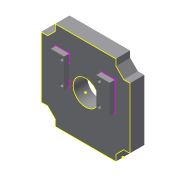
# Autodesk Inventor part: 20_Cube_Insert_RaspiCam_v3
Saved by Autodesk Inventor 2019.4 (Build 234330000, 330)
## iProperties
Created: 2019-07-01
Part Number: 20_Cube_Insert_RaspiCam_v3
Material: Generic
Document SubType Name: Modeling
Designer: diederichbenedict
Density: 1 g/cm^3
Appearance: Default
Author: diederichbenedict
Autodesk Inventor part; units mm, degrees
ref_plane "YZ Plane" through (0, 0, 0) normal (1, 0, 0) x (0, 1, 0)
ref_plane "Work Plane1" through (0, 0, 10) normal (0, 0, 1) x (1, 0, 0)
sketch "Sketch1" plane through (0, 0, 10) normal (0, 0, 1) x (1, 0, 0)
  line L0 (-4.0299, -0.3538) -> (-2.2322, 1.4439) construction
  arc A0 (-1.4439, 2.2322) -> (-2.2322, 1.4439) centre (-0.9299, 0.9299) ccw construction
  line L1 (-1.4439, 2.2322) -> (0.3538, 4.0299) construction
  line L2 (-37.8299, 42.2137) -> (-37.8299, 45.8299) construction
  line L3 (-37.8299, 45.8299) -> (-4.0299, 45.8299) construction
  line L4 (-4.0299, 45.8299) -> (-4.0299, 42.2137) construction
  line L5 (-4.0299, 4.0299) -> (0.3538, 4.0299) projected
  circle A1 centre (-20.9299, 20.9299) radius 17.5 projected
  line L6 (-20.9299, 58.9723) -> (17.1124, 20.9299) construction
  line L7 (17.1124, 20.9299) -> (-20.9299, -17.1124) construction
  line L8 (-20.9299, -17.1124) -> (-58.9723, 20.9299) construction
  line L9 (-58.9723, 20.9299) -> (-20.9299, 58.9723) construction
  line L10 (-20.9299, 58.9723) -> (-20.9299, -17.1124) construction
  line L11 (17.1124, 20.9299) -> (-58.9723, 20.9299) construction
  line L12 (-20.9299, 58.9723) -> (32.8701, 58.9723) construction
  line L13 (-43.4299, 43.4299) -> (1.5701, 43.4299) construction
  line L14 (1.5701, 43.4299) -> (1.5701, -1.5701) construction
  line L15 (1.5701, -1.5701) -> (-43.4299, -1.5701) construction
  line L16 (-43.4299, -1.5701) -> (-43.4299, 43.4299) construction
  line L17 (-43.4299, 43.4299) -> (1.5701, -1.5701) construction
  line L18 (1.5701, 43.4299) -> (-43.4299, -1.5701) construction
  line L19 (-43.4299, 5.3876) -> (-43.4299, 36.4723)
  line L20 (-43.4299, 36.4723) -> (-36.4723, 43.4299)
  line L21 (-36.4723, 43.4299) -> (-5.3876, 43.4299)
  line L22 (-5.3876, 43.4299) -> (1.5701, 36.4723)
  line L23 (1.5701, 36.4723) -> (1.5701, 5.3876)
  line L24 (1.5701, 5.3876) -> (-5.3876, -1.5701)
  line L25 (-5.3876, -1.5701) -> (-36.4723, -1.5701)
  line L26 (-36.4723, -1.5701) -> (-43.4299, 5.3876)
  line L27 (-4.0299, 42.2137) -> (-37.8299, 42.2137) projected
  line L28 (-4.0299, -0.3538) -> (-4.0299, 4.0299) projected
  circle A2 centre (-20.9299, 20.9299) radius 7.0417
  point P0 (-37.8299, 4.0299)
  dimension "d18" = 53.8
  dimension "d19" = 45
  dimension "d20" = 53.8
  dimension "d21" = 45
  dimension "d22" = 45
  constraints: 42 end point, 15 point on line, 5 midpoint, 4 parallel, 3 perpendicular, 2 horizontal, 1 centre point, 1 coincident, 1 equal length
  measures "d18" distance of L6.start L6.end
  measures "d19" angle of L6 L12
  measures "d20" distance of L6.end L7.end
  measures "d21" distance of L14.end L15.end
  measures "d22" distance of L13.end L14.end
extrude "Extrusion1" add sketch "Sketch1" along normal blind 8 contours L28 L24 L25 L26 L19 L20 L27 L22 L23 L5 | L5 L24 L28 | L27 L20 L21 L22 | A1
sketch "Sketch3" plane through (0, 0, 10) normal (0, 0, -1) x (-1, 0, 0)
  line L0 (37.8299, -0.4701) -> (37.8299, 4.0299) construction
  line L1 (4.0299, 4.0299) -> (4.0299, -0.4701) construction
  line L2 (37.8299, -0.4701) -> (37.8299, 1.1886) construction
  line L3 (4.0299, -3.9701) -> (4.0299, -0.3538) construction
  line L4 (45.8299, 4.0299) -> (42.2137, 4.0299) construction
  line L5 (-0.3538, 4.0299) -> (-3.9701, 4.0299) construction
  line L6 (-3.9701, 37.8299) -> (-0.3538, 37.8299) construction
  line L7 (4.0299, 42.2137) -> (4.0299, 45.8299) construction
  line L8 (37.8299, 45.8299) -> (37.8299, 42.2137) construction
  line L9 (42.2137, 37.8299) -> (45.8299, 37.8299) construction
  line L10 (37.8299, 37.7299) -> (45.8299, 37.7299)
  line L11 (45.8299, 37.7299) -> (45.8299, 4.1299)
  line L12 (45.8299, 4.1299) -> (37.8299, 4.1299)
  line L13 (37.8299, 4.1299) -> (37.8299, 37.7299)
  line L14 (37.7299, 4.0299) -> (4.1299, 4.0299)
  line L15 (4.1299, 4.0299) -> (4.1299, -3.9701)
  line L16 (4.1299, -3.9701) -> (37.7299, -3.9701)
  line L17 (37.7299, -3.9701) -> (37.7299, 4.0299)
  line L18 (4.0299, 4.1299) -> (-3.9701, 4.1299)
  line L19 (-3.9701, 4.1299) -> (-3.9701, 37.7299)
  line L20 (-3.9701, 37.7299) -> (4.0299, 37.7299)
  line L21 (4.0299, 37.7299) -> (4.0299, 4.1299)
  line L22 (4.1299, 37.8299) -> (37.7299, 37.8299)
  line L23 (37.7299, 37.8299) -> (37.7299, 45.8299)
  line L24 (37.7299, 45.8299) -> (4.1299, 45.8299)
  line L25 (4.1299, 45.8299) -> (4.1299, 37.8299)
  point P0 (0, 0)
  dimension "d23" = 0.1
  dimension "d24" = 0.1
  dimension "d25" = 0.1
  dimension "d26" = 0.1
  dimension "d27" = 0.1
  constraints: 32 end point, 8 parallel, 4 horizontal, 4 perpendicular, 3 point on line
  measures "d23" distance between parallel lines of L8 L23
  measures "d24" distance between parallel lines of L7 L25
  measures "d25" distance between parallel lines of L6 L20
  measures "d26" distance between parallel lines of L5 L18
  measures "d27" distance between parallel lines of L1 L15
extrude "Extrusion3" add sketch "Sketch3" against normal up to surface (8 mm away)
sketch "Sketch4" plane through (0, 0, 18) normal (0, 0, 1) x (1, 0, 0)
  line L0 (-33.4299, 35.4299) -> (-33.4299, 11.4299) construction
  line L1 (-33.4299, 11.4299) -> (-8.4299, 11.4299) construction
  line L2 (-8.4299, 11.4299) -> (-8.4299, 35.4299) construction
  line L3 (-8.4299, 35.4299) -> (-33.4299, 35.4299) construction
  circle A0 centre (-10.4299, 33.4299) radius 1.05 construction
  circle A1 centre (-10.4299, 20.9299) radius 1.05 construction
  circle A2 centre (-31.4299, 20.9299) radius 1.05 construction
  circle A3 centre (-31.4299, 33.4299) radius 1.05 construction
  line L4 (-15.4299, 29.8299) -> (-12.4299, 29.8299) construction
  line L5 (-15.4299, 31.8299) -> (-15.4299, 29.8299) construction
  line L6 (-12.4299, 31.8299) -> (-15.4299, 31.8299) construction
  line L7 (-12.4299, 29.8299) -> (-12.4299, 31.8299) construction
  line L8 (-8.4299, 35.4299) -> (-11.9299, 35.4299)
  line L9 (-11.9299, 35.4299) -> (-11.9299, 19.4299)
  line L10 (-11.9299, 19.4299) -> (-8.4299, 19.4299)
  line L11 (-8.4299, 19.4299) -> (-8.4299, 35.4299)
  line L12 (-33.4299, 35.4299) -> (-29.9299, 35.4299)
  line L13 (-29.9299, 35.4299) -> (-29.9299, 19.4299)
  line L14 (-29.9299, 19.4299) -> (-33.4299, 19.4299)
  line L15 (-33.4299, 19.4299) -> (-33.4299, 35.4299)
  line L16 (-33.4299, 35.4299) -> (-37.4299, 35.4299)
  line L17 (-37.4299, 35.4299) -> (-37.4299, 19.4299)
  line L18 (-37.4299, 19.4299) -> (-33.4299, 19.4299)
  line L19 (-33.4299, 19.4299) -> (-33.4299, 35.4299)
  line L20 (-8.4299, 35.4299) -> (-4.4299, 35.4299)
  line L21 (-4.4299, 35.4299) -> (-4.4299, 19.4299)
  line L22 (-4.4299, 19.4299) -> (-8.4299, 19.4299)
  line L23 (-8.4299, 19.4299) -> (-8.4299, 35.4299)
  point P0 (0, 0)
  dimension "d30" = 3.5
  dimension "d31" = 16
  dimension "d32" = 3.5
  dimension "d37" = 4
  dimension "d38" = 4
  constraints: 32 end point, 8 parallel, 4 horizontal, 4 perpendicular, 2 point on line
  measures "d30" distance of L10.end L9.end
  measures "d31" distance of L9.end L8.end
  measures "d32" distance of L13.end L14.end
  measures "d37" distance of L18.end L17.end
  measures "d38" distance of L21.end L22.end
ref_plane "Work Plane3" through (-33.4299, 11.4299, 16.4) normal (0, 0, -1) x (0, 1, 0)
extrude "Extrusion4" add sketch "Sketch4" along normal blind 3
sketch "Sketch5" plane through (-11.9299, 35.4299, 21) normal (0, 0, 1) x (1, 0, 0)
  circle A0 centre (1.5, -14.5) radius 1.05 projected
  circle A1 centre (1.5, -2) radius 1.05 projected
  circle A2 centre (-19.5, -2) radius 1.05 projected
  circle A3 centre (-19.5, -14.5) radius 1.05 projected
  point P0 (11.9299, -35.4299)
extrude "Extrusion5" cut sketch "Sketch5" against normal through all
sketch "Skizze12" plane through (0, 0, 10) normal (0, 0, -1) x (-1, 0, 0)
  line L0 (-0.3124, 4.1299) -> (4.1299, -0.3124) projected
  line L1 (4.1299, -0.3124) -> (4.1299, -3.9701) projected
  line L2 (4.1299, -3.9701) -> (37.7299, -3.9701) construction
  line L3 (37.7299, -3.9701) -> (37.7299, -0.3124) projected
  line L4 (37.7299, -0.3124) -> (42.1723, 4.1299) projected
  line L5 (45.8299, 4.1299) -> (42.1723, 4.1299) projected
  line L6 (45.8299, 37.7299) -> (45.8299, 4.1299) construction
  line L7 (42.1723, 37.7299) -> (45.8299, 37.7299) projected
  line L8 (42.1723, 37.7299) -> (37.7299, 42.1723) projected
  line L9 (37.7299, 42.1723) -> (37.7299, 45.8299) projected
  line L10 (37.7299, 45.8299) -> (4.1299, 45.8299) construction
  line L11 (4.1299, 45.8299) -> (4.1299, 42.1723) projected
  line L12 (4.1299, 42.1723) -> (-0.3124, 37.7299) projected
  line L13 (-3.9701, 37.7299) -> (-0.3124, 37.7299) projected
  line L14 (-3.9701, 4.1299) -> (-3.9701, 37.7299) construction
  line L15 (-0.3124, 4.1299) -> (-3.9701, 4.1299) projected
  circle A0 centre (20.9299, 20.9299) radius 7.0417 construction
  line L16 (37.9299, -4.1701) -> (3.9299, -4.1701) construction
  line L17 (3.9299, -4.1701) -> (3.9299, -0.3953)
  line L18 (3.9299, -0.3953) -> (-0.3953, 3.9299)
  line L19 (-0.3953, 3.9299) -> (-4.1701, 3.9299)
  line L20 (-4.1701, 3.9299) -> (-4.1701, 37.9299) construction
  line L21 (-4.1701, 37.9299) -> (-0.3953, 37.9299)
  line L22 (-0.3953, 37.9299) -> (3.9299, 42.2551)
  line L23 (3.9299, 42.2551) -> (3.9299, 46.0299)
  line L24 (3.9299, 46.0299) -> (37.9299, 46.0299) construction
  line L25 (37.9299, 46.0299) -> (37.9299, 42.2551)
  line L26 (37.9299, 42.2551) -> (42.2551, 37.9299)
  line L27 (42.2551, 37.9299) -> (46.0299, 37.9299)
  line L28 (46.0299, 37.9299) -> (46.0299, 3.9299) construction
  line L29 (46.0299, 3.9299) -> (42.2551, 3.9299)
  line L30 (42.2551, 3.9299) -> (37.9299, -0.3953)
  line L31 (37.9299, -0.3953) -> (37.9299, -4.1701)
  line L32 (-3.9701, 37.7299) -> (-3.9701, 37.9299)
  line L33 (37.7299, 45.8299) -> (4.1299, 45.8299) projected
  line L34 (4.1299, 45.8299) -> (3.9299, 45.8299)
  line L35 (37.7299, 45.8299) -> (37.9299, 45.8299)
  line L36 (45.8299, 37.7299) -> (45.8299, 37.9299)
  line L37 (45.8299, 4.1299) -> (45.8299, 3.9299)
  line L38 (37.7299, -3.9701) -> (37.9299, -3.9701)
  line L39 (4.1299, -3.9701) -> (3.9299, -3.9701)
  line L40 (-3.9701, 4.1299) -> (-3.9701, 3.9299)
  point P0 (0, 0)
  dimension "d65" = 0.2
  constraints: 48 end point, 13 point on line, 2 perpendicular, 1 vertical, 15 other
  measures "d65" distance between parallel lines of L2 L16
extrude "IM_offset" add sketch "Skizze12" against normal up to surface (8 mm away)
sketch "Sketch13" plane through (0, 0, 18) normal (0, 0, 1) x (1, 0, 0)
  line L0 (3.9701, 37.9299) -> (3.9701, 3.9299) projected
  line L1 (0.3953, 37.9299) -> (3.9701, 37.9299) projected
  line L2 (-3.9299, 42.2551) -> (0.3953, 37.9299) projected
  line L3 (-3.9299, 45.8299) -> (-3.9299, 42.2551) projected
  line L4 (-37.9299, 45.8299) -> (-3.9299, 45.8299) projected
  line L5 (-37.9299, 42.2551) -> (-37.9299, 45.8299) projected
  line L6 (-42.2551, 37.9299) -> (-37.9299, 42.2551) projected
  line L7 (-45.8299, 37.9299) -> (-42.2551, 37.9299) projected
  line L8 (-45.8299, 3.9299) -> (-45.8299, 37.9299) projected
  line L9 (-42.2551, 3.9299) -> (-45.8299, 3.9299) projected
  line L10 (-37.9299, -0.3953) -> (-42.2551, 3.9299) projected
  line L11 (-37.9299, -3.9701) -> (-37.9299, -0.3953) projected
  line L12 (-3.9299, -3.9701) -> (-37.9299, -3.9701) projected
  line L13 (-3.9299, -0.3953) -> (-3.9299, -3.9701) projected
  line L14 (0.3953, 3.9299) -> (-3.9299, -0.3953) projected
  line L15 (3.9701, 3.9299) -> (0.3953, 3.9299) projected
  circle A0 centre (-20.9299, 20.9299) radius 7.0417 projected
  line L16 (-33.2963, 30.7242) -> (-29.9299, 30.7242) projected
  line L17 (-29.9299, 30.7242) -> (-29.9299, 35.4299) projected
  line L18 (-29.9299, 35.4299) -> (-37.4299, 35.4299) projected
  line L19 (-37.4299, 35.4299) -> (-37.4299, 19.4299) projected
  line L20 (-37.4299, 19.4299) -> (-29.9299, 19.4299) projected
  line L21 (-29.9299, 19.4299) -> (-29.9299, 22.7242) projected
  line L22 (-29.9299, 22.7242) -> (-33.2963, 22.7242) projected
  line L23 (-33.2963, 22.7242) -> (-33.2963, 30.7242) projected
  circle A1 centre (-31.4299, 33.4299) radius 1.05 projected
  circle A2 centre (-31.4299, 20.9299) radius 1.05 projected
  line L24 (-8.2963, 22.7242) -> (-11.9299, 22.7242) projected
  line L25 (-11.9299, 22.7242) -> (-11.9299, 19.4299) projected
  line L26 (-11.9299, 19.4299) -> (-4.4299, 19.4299) projected
  line L27 (-4.4299, 19.4299) -> (-4.4299, 35.4299) projected
  line L28 (-4.4299, 35.4299) -> (-11.9299, 35.4299) projected
  line L29 (-11.9299, 35.4299) -> (-11.9299, 30.7242) projected
  line L30 (-11.9299, 30.7242) -> (-8.2963, 30.7242) projected
  line L31 (-8.2963, 30.7242) -> (-8.2963, 22.7242) projected
  circle A3 centre (-10.4299, 20.9299) radius 1.05 projected
  circle A4 centre (-10.4299, 33.4299) radius 1.05 projected
  point P0 (0, 0)
body "Solid1"
